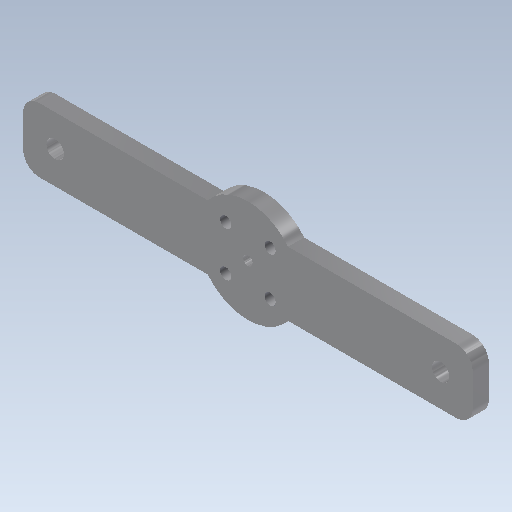
# Autodesk Inventor part: rudder_horn
Saved by Autodesk Inventor 2020 (Build 240168000, 168)
## iProperties
Created: 2016-11-14
Part Number: rudder_horn
Material: Generic
Document SubType Name: Sheet Metal
Designer: jous
Density: 1 g/cm^3
Appearance: Default
Sheet Metal Rule: Default
Mass: 14.4707 g
Surface Area: 78.2231 cm^2
Volume: 14.4707 cm^3
Author: jous
Autodesk Inventor part; units mm, degrees
ref_plane "YZ Plane" through (0, 0, 0) normal (1, 0, 0) x (0, 1, 0)
ref_plane "XZ Plane" through (0, 0, 0) normal (0, 1, 0) x (-1, 0, 0)
ref_plane "XY Plane" through (0, 0, 0) normal (0, 0, 1) x (1, 0, 0)
sketch "Sketch1" plane through (0, 0, 0) normal (0, 0, 1) x (1, 0, 0)
  line L0 (-70, -10) -> (70, -10)
  line L1 (70, -10) -> (70, 10)
  line L2 (70, 10) -> (-70, 10)
  line L3 (-70, 10) -> (-70, -10)
  line L4 (-70, -10) -> (70, 10) construction
  line L5 (70, -10) -> (-70, 10) construction
  circle A0 centre (0, 0) radius 16
  line L6 (-73.4722, 0) -> (96.5278, 0) construction
  circle A1 centre (-60, 0) radius 2.75
  line L7 (0, 0) -> (0, 31) construction
  circle A2 centre (60, 0) radius 2.75
  circle A3 centre (0, 0) radius 1.5
  circle A4 centre (-6.9148, 6.9148) radius 1.7526
  line L8 (0, 0) -> (-14.5685, 14.5685) construction
  circle A5 centre (-6.9148, -6.9148) radius 1.7526
  circle A6 centre (6.9148, -6.9148) radius 1.7526
  circle A7 centre (6.9148, 6.9148) radius 1.7526
  point P0 (0, 0)
  dimension "d0" = 140
  dimension "d1" = 20
  dimension "d4" = 32
  dimension "d5" = 5.5
  dimension "d6" = 10
  dimension "d10" = 3
  dimension "d11" = 3.5052
  dimension "d12" = 45
  dimension "d13" = 6.9148
  dimension "d16" = 360
  constraints: 18 end point, 8 centre point, 3 midpoint, 3 point on line, 2 coincident, 2 equal length, 2 perpendicular, 1 parallel, 1 symmetric about line, 1 vertical, 10 other
  measures "d0" distance of L2.end L1.end
  measures "d1" distance of L1.end L0.end
  measures "d4" diameter of A0
  measures "d5" diameter of A1
  measures "d6" distance from line of A1.centre L3
  measures "d10" diameter of A3
  measures "d11" diameter of A4
  measures "d12" angle of L6 L8
  measures "d13" distance from line of L6 A4.centre
extrude "Extrusion1" add sketch "Sketch1" along normal blind 5 contours L3 L2 A0 L0 | A0 L2 L0 | L0 A0 | A0 L2 L1 L0 | A0 L2 | A1 | A2 | A3 | A4 | A5 | A6 | A7
extrude "Extrusion2" cut sketch "Sketch1" along normal through all contours A1 | A2 | A3 | A4 | A5 | A6 | A7
fillet "Fillet1" radius 5 4 edges at (70, -10, 2.5) (70, 10, 2.5) (-70, -10, 2.5) (-70, 10, 2.5)
equation "\"BendRadius\" = Thickness"
equation "\"BendReliefWidth\" = Thickness"
equation "\"BendReliefDepth\" = 0.5 * Thickness"
equation "\"CornerReliefSize\" = 4 * Thickness"
equation "\"MinimumRemnant\" = 2 * Thickness"
equation "\"TransitionRadius\" = BendRadius"
equation "\"JacobiRadiusSize\" = Thickness"
equation "\"GapSize\" = Thickness"
equation "\"Thickness\" = 0.5"
body "Solid1"
